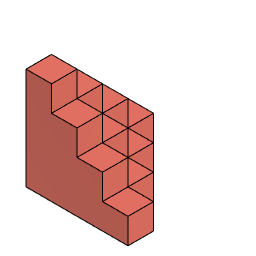
Cubes (Autodesk Fusion 360 design; units mm, degrees)
Autodesk Fusion 360 part; units mm, degrees
sketch "Sketch1" plane through (0, 0, 0) normal (0, 0, 1) x (1, 0, 0)
  line L0 (0, 0) -> (20, 0)
  line L1 (20, 0) -> (20, 20)
  line L2 (20, 20) -> (0, 20)
  line L3 (0, 20) -> (0, 0)
  dimension "d1" = 20
  dimension "d2" = 20
  constraint horizontal L0
  constraint vertical L1
  constraint horizontal L2
  constraint vertical L3
  constraint coincident L0.start L3.end
  measures "d1" distance of L0.start L0.end
  measures "d2" distance of L0.start L2.end
extrude "Extrude1" add sketch "Sketch1" along normal blind 20 makes body 1
copy_body "CopyPasteBodies1" bodies 1 makes body 2
move_body "Move1" bodies 2 to x (1, 0, 0) y (0, 1, 0) z (0, 0, 1) at (20, 0, 0)
copy_body "CopyPasteBodies2" bodies 1 makes body 3
move_body "Move2" bodies 3 to x (1, 0, 0) y (0, 1, 0) z (0, 0, 1) at (0, 20, 0)
copy_body "CopyPasteBodies3" bodies 1 makes body 4
move_body "Move3" bodies 4 to x (1, 0, 0) y (0, 1, 0) z (0, 0, 1) at (40, 0, 0)
copy_body "CopyPasteBodies4" bodies 1 makes body 5
move_body "Move4" bodies 5 to x (1, 0, 0) y (0, 1, 0) z (0, 0, 1) at (0, 40, 0)
copy_body "CopyPasteBodies5" bodies 1 makes body 6
move_body "Move5" bodies 6 to x (1, 0, 0) y (0, 1, 0) z (0, 0, 1) at (20, 20, 0)
copy_body "CopyPasteBodies6" bodies 1 makes body 7
move_body "Move6" bodies 7 to x (1, 0, 0) y (0, 1, 0) z (0, 0, 1) at (60, 0, 0)
copy_body "CopyPasteBodies7" bodies 1 makes body 8
move_body "Move7" bodies 8 to x (1, 0, 0) y (0, 1, 0) z (0, 0, 1) at (0, 60, 0)
copy_body "CopyPasteBodies8" bodies 1 makes body 9
move_body "Move8" bodies 9 to x (1, 0, 0) y (0, 1, 0) z (0, 0, 1) at (20, 40, 0)
copy_body "CopyPasteBodies9" bodies 1 makes body 10
move_body "Move9" bodies 10 to x (1, 0, 0) y (0, 1, 0) z (0, 0, 1) at (40, 20, 0)
copy_body "CopyPasteBodies10" bodies 1 makes body 11
move_body "Move10" bodies 11 to x (1, 0, 0) y (0, 1, 0) z (0, 0, 1) at (0, 0, 20)
copy_body "CopyPasteBodies11" bodies 1 makes body 12
move_body "Move11" bodies 12 to x (1, 0, 0) y (0, 1, 0) z (0, 0, 1) at (0, 0, 40)
copy_body "CopyPasteBodies12" bodies 1 makes body 13
move_body "Move12" bodies 13 to x (1, 0, 0) y (0, 1, 0) z (0, 0, 1) at (0, 0, 60)
copy_body "CopyPasteBodies13" bodies 1 makes body 14
move_body "Move13" bodies 14 to x (1, 0, 0) y (0, 1, 0) z (0, 0, 1) at (0, 20, 20)
copy_body "CopyPasteBodies14" bodies 1 makes body 15
move_body "Move14" bodies 15 to x (1, 0, 0) y (0, 1, 0) z (0, 0, 1) at (0, 40, 20)
copy_body "CopyPasteBodies15" bodies 1 makes body 16
move_body "Move15" bodies 16 to x (1, 0, 0) y (0, 1, 0) z (0, 0, 1) at (20, 20, 20)
copy_body "CopyPasteBodies16" bodies 1 makes body 17
move_body "Move16" bodies 17 to x (1, 0, 0) y (0, 1, 0) z (0, 0, 1) at (20, 0, 20)
copy_body "CopyPasteBodies17" bodies 1 makes body 18
move_body "Move17" bodies 18 to x (1, 0, 0) y (0, 1, 0) z (0, 0, 1) at (40, 0, 20)
copy_body "CopyPasteBodies18" bodies 1 makes body 19
move_body "Move18" bodies 19 to x (1, 0, 0) y (0, 1, 0) z (0, 0, 1) at (20, 0, 40)
copy_body "CopyPasteBodies19" bodies 1 makes body 20
move_body "Move19" bodies 20 to x (1, 0, 0) y (0, 1, 0) z (0, 0, 1) at (0, 20, 40)
combine "Combine1" operation add target body 14 tool bodies 7 4 15 11 20 12 16 17 8 5 19 18 2 10 9 6 3 1 13
shell "Shell1" thickness 4 removed faces 1 at (33.3333, 20, 0) on bodies 14
component "cubes" placed x (1, 0, 0) y (0, 1, 0) z (0, 0, 1) at (0, 0, 0)
